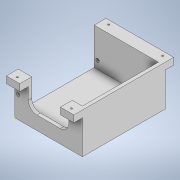
# Autodesk Inventor part: encaixe2 mouse
Saved by Autodesk Inventor 2022 (Build 260153000, 153)
## iProperties
Created: 2024-03-11
Part Number: encaixe2 mouse
Material: Generic
Document SubType Name: Modeling
Designer: admin
Density: 1 g/cm^3
Appearance: Default
Author: admin
Autodesk Inventor part; units mm, degrees
ref_plane "YZ Plane" through (0, 0, 0) normal (1, 0, 0) x (0, 1, 0)
ref_plane "XZ Plane" through (0, 0, 0) normal (0, 1, 0) x (-1, 0, 0)
ref_plane "XY Plane" through (0, 0, 0) normal (0, 0, 1) x (1, 0, 0)
sketch "Sketch1" plane through (0, 0, 0) normal (0, 1, 0) x (-1, 0, 0)
  line L0 (0, 0) -> (40, 0)
  line L1 (40, 0) -> (40, -49)
  line L2 (40, -49) -> (0, -49)
  line L3 (0, -49) -> (0, 0)
  dimension "d0" = 40
  dimension "d1" = 49
  constraints: 8 end point, 2 parallel, 1 horizontal, 1 perpendicular
  measures "d0" distance of L1.end L2.end
  measures "d1" distance of L0.end L1.end
extrude "Extrusion1" add sketch "Sketch1" along normal blind 24
sketch "Sketch2" plane through (0, 24, 0) normal (0, 1, 0) x (1, 0, 0)
  line L0 (0, 0) -> (0, 49) projected
  line L1 (0, 49) -> (-40, 49) projected
  line L2 (0, 0) -> (-2, 0)
  line L3 (-2, 0) -> (-2, 49)
  line L4 (-2, 49) -> (0, 49)
  line L5 (0, 49) -> (0, 0)
  line L6 (-40, 49) -> (-40, 0) projected
  line L7 (-40, 0) -> (-38, 0)
  line L8 (-38, 0) -> (-38, 49)
  line L9 (-38, 49) -> (-40, 49)
  line L10 (-40, 49) -> (-40, 0)
  line L11 (0, 0) -> (-40, 0)
  line L12 (-40, 0) -> (-40, 2)
  line L13 (-40, 2) -> (0, 2)
  line L14 (0, 2) -> (0, 0)
  line L15 (0, 49) -> (-40, 49)
  line L16 (-40, 49) -> (-40, 47)
  line L17 (-40, 47) -> (0, 47)
  line L18 (0, 47) -> (0, 49)
  line L19 (-2, 47) -> (-38, 47)
  line L20 (-38, 47) -> (-38, 2)
  line L21 (-38, 2) -> (-2, 2)
  line L22 (-2, 2) -> (-2, 47)
  point P0 (-38, 47)
  dimension "d4" = 2
  dimension "d5" = 2
  dimension "d6" = 2
  dimension "d7" = 2
  constraints: 40 end point, 10 parallel, 8 point on line, 5 horizontal, 5 perpendicular
  measures "d4" distance of L3.end L4.end
  measures "d5" distance of L9.end L8.end
  measures "d6" distance of L11.end L12.end
  measures "d7" distance of L16.end L15.end
extrude "Extrusion2" cut sketch "Sketch2" against normal blind 21.75 contours L13 L8 L17 L3
sketch "Sketch3" plane through (-40, 0, 0) normal (0, 0, 1) x (1, 0, 0)
  line L0 (0, 24) -> (40, 24) projected
  line L1 (0, 0) -> (40, 0) projected
  line L2 (0, 24) -> (8, 24)
  line L3 (8, 24) -> (8, 0)
  line L4 (8, 0) -> (0, 0)
  line L5 (0, 0) -> (0, 24)
  line L6 (0, 0) -> (0, 24) projected
  line L7 (40, 0) -> (40, 24) projected
  line L8 (0, 0) -> (40, 0)
  line L9 (40, 0) -> (40, 8)
  line L10 (40, 8) -> (0, 8)
  line L11 (0, 8) -> (0, 0)
  line L12 (38, 24) -> (2, 24) projected
  line L13 (40, 0) -> (32, 0)
  line L14 (32, 0) -> (32, 24)
  line L15 (32, 24) -> (40, 24)
  line L16 (40, 24) -> (40, 0)
  line L17 (8, 24) -> (32, 24)
  line L18 (32, 24) -> (32, 8)
  line L19 (32, 8) -> (8, 8)
  line L20 (8, 8) -> (8, 24)
  point P0 (8, 8)
  dimension "d10" = 8
  dimension "d11" = 8
  dimension "d12" = 8
  constraints: 32 end point, 8 parallel, 5 point on line, 4 horizontal, 4 perpendicular
  measures "d10" distance of L3.end L4.end
  measures "d11" distance of L9.end L8.end
  measures "d12" distance of L14.end L15.end
extrude "Extrusion3" cut sketch "Sketch3" against normal blind 21 contours L0 L14 L10 L3
fillet "Fillet1" radius 5 2 edges at (-32, 8, -1) (-8, 8, -1)
sketch "Sketch4" plane through (-40, 0, 0) normal (0, 0, 1) x (1, 0, 0)
  line L0 (0, 0) -> (0, 24) projected
  line L1 (8, 13) -> (8, 24) projected
  line L2 (0, 24) -> (8, 24)
  line L3 (8, 24) -> (8, 20)
  line L4 (8, 20) -> (0, 20)
  line L5 (0, 20) -> (0, 24)
  line L6 (32, 24) -> (40, 24) projected
  line L7 (32, 13) -> (32, 24) projected
  line L8 (40, 24) -> (32, 24)
  line L9 (32, 24) -> (32, 20)
  line L10 (32, 20) -> (40, 20)
  line L11 (40, 20) -> (40, 24)
  point P0 (40, 0)
  point P1 (0, 20)
  dimension "d16" = 4
  dimension "d17" = 4
  constraints: 16 end point, 4 parallel, 2 horizontal, 2 perpendicular, 2 point on line
  measures "d16" distance of L2.end L3.end
  measures "d17" distance of L9.end L8.end
extrude "Extrusion4" add sketch "Sketch4" along normal blind 5
sketch "Sketch5" plane through (0, 0, -49) normal (0, 0, -1) x (-1, 0, 0)
  line L0 (40, 0) -> (40, 24) projected
  line L1 (0, 24) -> (40, 24)
  line L2 (40, 24) -> (40, 20)
  line L3 (40, 20) -> (0, 20)
  line L4 (0, 20) -> (0, 24)
  point P0 (0, 0)
  dimension "d20" = 4
  constraints: 8 end point, 2 parallel, 1 horizontal, 1 perpendicular, 1 point on line
  measures "d20" distance of L1.end L2.end
extrude "Extrusion5" add sketch "Sketch5" along normal blind 5
sketch "Sketch6" plane through (-2, 24, -47) normal (-1, 0, 0) x (0, 0, 1)
  line L0 (0, 0) -> (0, -21.75) projected
  line L1 (0, 0) -> (45, 0) projected
  line L2 (0, -21.75) -> (45, -21.75)
  line L3 (45, -21.75) -> (45, 0)
  line L4 (45, 0) -> (0, 0)
  line L5 (0, 0) -> (0, -21.75)
  point P0 (47, -24)
  constraints: 8 end point, 2 parallel, 1 horizontal, 1 perpendicular
extrude "Extrusion6" cut sketch "Sketch6" along normal blind 50
sketch "Sketch10" plane through (0, 0, 0) normal (0, -1, 0) x (1, 0, 0)
  line L0 (-8, 5) -> (0, 5) projected
  line L1 (0, 5) -> (-4, 5)
  line L2 (-4, 5) -> (-4, 2.5)
  line L3 (-4, 2.5) -> (0, 2.5)
  line L4 (0, 2.5) -> (0, 5)
  circle A0 centre (-4, 2.5) radius 0.5
  line L5 (-40, 0) -> (-40, 5) projected
  line L6 (-40, 5) -> (-36, 5)
  line L7 (-36, 5) -> (-36, 2.5)
  line L8 (-36, 2.5) -> (-40, 2.5)
  line L9 (-40, 2.5) -> (-40, 5)
  circle A1 centre (-36, 2.5) radius 0.5
  line L10 (-40, 5) -> (-40, -54) projected
  line L11 (-40, -54) -> (-36, -54)
  line L12 (-36, -54) -> (-36, -51.5)
  line L13 (-36, -51.5) -> (-40, -51.5)
  line L14 (-40, -51.5) -> (-40, -54)
  circle A2 centre (-36, -51.5) radius 0.5
  line L15 (0, -54) -> (0, 5) projected
  line L16 (0, -54) -> (-4, -54)
  line L17 (-4, -54) -> (-4, -51.5)
  line L18 (-4, -51.5) -> (0, -51.5)
  line L19 (0, -51.5) -> (0, -54)
  circle A3 centre (-4, -51.5) radius 0.5
  point P0 (0, 0)
  point P1 (0, -47)
  dimension "d41" = 4
  dimension "d42" = 2.5
  dimension "d43" = 1
  dimension "d44" = 4
  dimension "d45" = 2.5
  dimension "d46" = 1
  dimension "d49" = 4
  dimension "d50" = 2.5
  dimension "d51" = 1
  dimension "d53" = 4
  dimension "d54" = 2.5
  dimension "d55" = 1
  constraints: 32 end point, 8 parallel, 4 centre point, 4 coincident, 4 horizontal, 4 perpendicular
  measures "d41" distance of L3.end L2.end
  measures "d42" distance of L2.end L1.end
  measures "d43" diameter of A0
  measures "d44" distance of L7.end L8.end
  measures "d45" distance of L6.end L7.end
  measures "d46" diameter of A1
  measures "d49" distance of L13.end L12.end
  measures "d50" distance of L12.end L11.end
  measures "d51" diameter of A2
  measures "d53" distance of L17.end L18.end
  measures "d54" distance of L16.end L17.end
  measures "d55" diameter of A3
extrude "Extrusion10" cut sketch "Sketch10" against normal blind 30 contours A0 L3 L2 | L2 L3 A0 | A3 L17 L18 | L18 L17 A3 | A1 L7 L8 | L8 L7 A1 | A2 L12 L13 | L13 L12 A2
sketch "Sketch12" plane through (-40, 0, 0) normal (0, 0, 1) x (1, 0, 0)
  line L0 (40, 20) -> (36.5, 20)
  line L1 (0, 20) -> (2, 20)
  line L2 (2, 20) -> (2, 13)
  line L3 (2, 13) -> (0, 13)
  line L4 (0, 13) -> (0, 20)
  circle A0 centre (2, 13) radius 1
  point P0 (40, 0)
  dimension "d76" = 2
  dimension "d77" = 7
  dimension "d78" = 2
  constraints: 10 end point, 2 horizontal, 2 parallel, 1 centre point, 1 coincident, 1 perpendicular
  measures "d76" distance of L2.end L3.end
  measures "d77" distance of L1.end L2.end
  measures "d78" diameter of A0
extrude "Extrusion12" cut sketch "Sketch12" against normal blind 5 contours A0 L3 L2 | L2 L3 A0
sketch "Sketch14" plane through (0, 0, -49) normal (0, 0, -1) x (-1, 0, 0)
  line L0 (0, 0) -> (40, 0) projected
  line L1 (40, 0) -> (38, 0)
  line L2 (38, 0) -> (38, 7)
  line L3 (38, 7) -> (40, 7)
  line L4 (40, 7) -> (40, 0)
  circle A0 centre (38, 7) radius 1
  dimension "d79" = 2
  dimension "d80" = 7
  dimension "d81" = 2
  constraints: 8 end point, 2 parallel, 1 centre point, 1 coincident, 1 horizontal, 1 perpendicular
  measures "d79" distance of L2.end L3.end
  measures "d80" distance of L1.end L2.end
  measures "d81" diameter of A0
extrude "Extrusion14" cut sketch "Sketch14" against normal blind 5 contours A0 L3 L2 | L2 L3 A0
sketch "Sketch15" plane through (-40, 0, -49) normal (-1, 0, 0) x (0, 0, 1)
  point P0 (49, 0)
body "Solid1"
